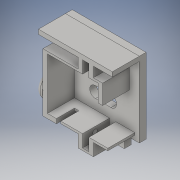
# Autodesk Inventor part: Hip_holder_bare_bone
Saved by Autodesk Inventor 2016 (Build 200138000, 138)
## iProperties
Created: 2018-07-11
Part Number: Hip_holder_bare_bone
Material: Generic
Document SubType Name: Modeling
Designer: Attila
Density: 1 g/cm^3
Appearance: Default
Author: Attila
Autodesk Inventor part; units mm, degrees
sketch "Sketch1" plane through (0, 0, 0) normal (0, 0, 1) x (1, 0, 0)
  line L0 (-20, -25) -> (20, -25)
  line L1 (20, -25) -> (20, 25)
  line L2 (20, 25) -> (-20, 25)
  line L3 (-20, 25) -> (-20, -25)
  line L4 (-20, -25) -> (20, 25) construction
  line L5 (20, -25) -> (-20, 25) construction
  point P0 (0, 0)
  dimension "Szelesseg" = 40
  dimension "Magassag" = 50
  constraints: 12 end point, 2 midpoint, 2 parallel, 1 horizontal, 1 perpendicular
  measures "Szelesseg" distance between parallel lines of L1 L3
  measures "Magassag" distance between parallel lines of L0 L2
extrude "Extrusion1" add sketch "Sketch1" along normal blind 3
sketch "Sketch12" plane through (0, 0, 3) normal (0, 0, 1) x (1, 0, 0)
  line L0 (9.3631, -13.3631) -> (5.2631, -13.3631)
  line L1 (5.2631, -13.3631) -> (5.2631, -18.8631)
  line L2 (2.4631, -17.3356) -> (2.4631, -13.3631)
  line L3 (-13.1369, -13.3631) -> (-13.1369, 9.5369)
  line L4 (-13.1369, 9.5369) -> (2.4631, 9.5369)
  line L5 (2.4631, 9.5369) -> (2.4631, 15.0369)
  line L6 (2.4631, 15.0369) -> (5.2631, 15.0369)
  line L7 (5.2631, 15.0369) -> (5.2631, 9.5369)
  line L8 (5.2631, 9.5369) -> (9.3631, 9.5369)
  line L9 (9.3631, 9.5369) -> (9.3631, 1.9369)
  line L10 (7.2631, -14.3631) -> (7.2631, -19.8631)
  line L11 (7.2631, -19.8631) -> (0.4631, -19.8631)
  line L12 (0.4631, -19.8631) -> (0.4631, -14.3631)
  line L13 (-15.1369, -15.3631) -> (-15.1369, 10.5369)
  line L14 (-15.1369, 10.5369) -> (0.4631, 10.5369)
  line L15 (0.4631, 10.5369) -> (0.4631, 15.0369)
  line L16 (7.2631, 15.0369) -> (7.2631, 10.5369)
  line L17 (7.2631, 10.5369) -> (11.3631, 10.5369)
  line L18 (11.3631, 10.5369) -> (11.3631, 3.6471)
  line L19 (7.2631, -14.3631) -> (13.6631, -14.3631)
  line L20 (13.6631, -14.3631) -> (13.6631, -13.3631)
  line L21 (13.6631, -13.3631) -> (9.3631, -13.3631)
  line L22 (-9.1369, -15.3631) -> (-9.1369, -13.3631)
  line L23 (-7.1369, -14.3631) -> (-7.1369, -13.3631)
  line L24 (0.4631, -14.3631) -> (-7.1369, -14.3631)
  line L25 (-9.1369, -15.3631) -> (-15.1369, -15.3631)
  line L26 (2.4631, -13.3631) -> (-7.1369, -13.3631)
  line L27 (-9.1369, -13.3631) -> (-13.1369, -13.3631)
  line L28 (18.3631, 23.3631) -> (18.3631, -23.3631) projected
  line L29 (18.3631, -23.3631) -> (-18.3631, -23.3631) projected
  line L30 (-18.3631, 23.3631) -> (18.3631, 23.3631) projected
  line L31 (2.4631, -17.3356) -> (2.4631, -18.8631)
  line L32 (-16.127, -21.127) -> (16.127, -21.127) projected
  line L33 (2.4631, -18.8631) -> (5.2631, -18.8631)
  line L34 (11.3631, 3.6471) -> (11.3631, 1.9369)
  line L35 (11.3631, 1.9369) -> (9.3631, 1.9369)
  line L36 (-9.1369, -14.3631) -> (-7.1369, -14.3631)
  line L37 (-9.1369, -13.3631) -> (-7.1369, -13.3631)
  line L38 (7.2631, 15.0369) -> (18.3631, 15.0369)
  line L39 (18.3631, 15.0369) -> (18.3631, 17.0369)
  line L40 (18.3631, 17.0369) -> (-18.3631, 17.0369)
  line L41 (-18.3631, 17.0369) -> (-18.3631, 15.0369)
  line L42 (-18.3631, 15.0369) -> (0.4631, 15.0369)
  line L43 (-18.3631, -23.3631) -> (-18.3631, 15.0369)
  line L44 (-18.3631, 17.0369) -> (-18.3631, 23.3631)
  line L45 (-17.1371, 15.0369) -> (-17.1371, 17.0369)
  line L46 (15.6631, 15.0369) -> (15.6631, 17.0369)
  point P0 (19.6785, 0.2929)
  dimension "d83" = 22.5
  dimension "d85" = 2.8
  dimension "d86" = 2.8
  dimension "d87" = 15.6
  dimension "d88" = 15.6
  dimension "d89" = 4.1
  dimension "d90" = 4.1
  dimension "d91" = 7.6
  dimension "d92" = 5.5
  dimension "d95" = 22.9
  dimension "d97" = 2
  dimension "d98" = 2
  dimension "d100" = 2
  dimension "d101" = 2
  dimension "d102" = 2
  dimension "d103" = 4.3
  dimension "d105" = 2
  dimension "d106" = 1
  dimension "d107" = 1
  dimension "d109" = 1
  dimension "d110" = 4
  dimension "d111" = 2
  dimension "d112" = 2
  dimension "d113" = 1
  dimension "d114" = 22.9
  dimension "d125" = 3.5
  dimension "d130" = 4.7
  dimension "d132" = 9
  dimension "d133" = 5.5
  dimension "d139" = 1
  dimension "d181" = 2
  dimension "d182" = 2
  dimension "d185" = 4.5
  dimension "d186" = 1.226
  dimension "d187" = 2.7
  constraints: 86 end point, 26 perpendicular, 12 point on line, 3 horizontal, 1 midpoint, 1 vertical
  measures "d83" distance between parallel lines of L9 L3
  measures "d85" distance between parallel lines of L5 L7
  measures "d86" distance between parallel lines of L2 L1
  measures "d87" distance of L3.end L4.end
  measures "d88" distance of L2.end L3.start
  measures "d89" distance of L8.end L7.end
  measures "d90" distance of L0.start L0.end
  measures "d91" distance of L8.end L9.end
  measures "d92" distance between parallel lines of L6 L8
  measures "d95" distance between parallel lines of L8 L0
  measures "d97" distance between parallel lines of L9 L18
  measures "d98" distance between parallel lines of L7 L16
  measures "d100" distance between parallel lines of L15 L5
  measures "d101" distance between parallel lines of L13 L3
  measures "d102" distance between parallel lines of L10 L1
  measures "d103" distance of L0.start L20.end
  measures "d105" distance between parallel lines of L12 L2
  measures "d106" distance between parallel lines of L17 L8
  measures "d107" distance between parallel lines of L14 L4
  measures "d109" distance between parallel lines of L0 L19
  measures "d110" distance between parallel lines of L3 L22
  measures "d111" distance between parallel lines of L22 L23
  measures "d112" distance between parallel lines of L27 L25
  measures "d113" distance between parallel lines of L26 L24
  measures "d114" distance between parallel lines of L4 L27
  measures "d125" distance between parallel lines of L29 L11
  measures "d130" distance from line of L20.end L28
  measures "d132" distance between parallel lines of L29 L19
  measures "d133" distance between parallel lines of L26 L33
  measures "d139" distance between parallel lines of L33 L11
  measures "d181" distance of L38.end L39.end
  measures "d182" distance of L40.end L41.end
  measures "d185" distance between parallel lines of L17 L38
  measures "d186" distance between parallel lines of L45 L41
  measures "d187" distance between parallel lines of L28 L46
ref_plane "Work Plane6" through (0, 0, 15) normal (0, 0, 1) x (1, 0, 0)
sketch "Sketch14" plane through (0, 0, 15) normal (0, 0, 1) x (1, 0, 0)
  line L0 (-9.1369, -14.3631) -> (0.4631, -14.3631) projected
  line L1 (-9.1369, -14.3631) -> (-9.1369, -13.3631)
  line L2 (-13.1369, -13.3631) -> (2.4631, -13.3631) projected
  line L3 (-7.1369, -13.3631) -> (-7.1369, -14.3631)
  point P0 (0, 0)
  dimension "d136" = 2
  constraints: 4 end point, 3 point on line, 1 parallel, 1 vertical
  measures "d136" distance between parallel lines of L3 L1
extrude "Extrusion5" cut sketch "Sketch14" against normal blind 8
ref_plane "Work Plane5" through (7.0131, -20.8631, 3) normal (1, 0, 0) x (0, 0, -1)
sketch "Sketch17" plane through (7.0131, -20.8631, 3) normal (1, 0, 0) x (0, 0, -1)
  line L0 (0, 0) -> (-12, 0) projected
  line L1 (0, 7.5) -> (-12, 7.5) projected
  line L2 (0, 6.5) -> (-12, 6.5) projected
  line L3 (-12, 7.5) -> (-12, 30.4) construction
  line L4 (-12, 18.95) -> (0, 18.95) construction
  line L5 (0, 37.9) -> (-12, 37.9) construction
  line L6 (0, 31.4) -> (-12, 31.4) construction
  point P0 (3, 20.8631)
  point P1 (-6.5, 5.5)
  point P2 (-6.5, 32.4)
  dimension "d144" = 1
  dimension "d145" = 18.95
  dimension "d146" = 1
  constraints: 2 end point, 1 midpoint, 1 perpendicular, 1 symmetric about line
  measures "d144" distance from line of point (-6.5, 5.5) L2
  measures "d145" distance between parallel lines of L5 L4
  measures "d146" distance from line of L6 point (-6.5, 32.4)
hole "Hole3" at (7.0131, -15.3631, 9.5) at (7.0131, 11.5369, 9.5) direction (-1, 0, 0) diameter 1.778 depth 8 tip angle 118
ref_plane "Work Plane1" through (-15.1369, -14.3631, 5) normal (-1, 0, 0) x (0, 0, 1)
sketch "Sketch18" plane through (-15.1369, -14.3631, 5) normal (-1, 0, 0) x (0, 0, 1)
  line L0 (9, 0) -> (0, 0) projected
  line L1 (-2, -9) -> (-2, 37.7262) projected
  circle A0 centre (3.9, 6.9) radius 3.6
  circle A1 centre (3.9, 6.9) radius 5.1
  point P0 (-5, 14.3631)
  dimension "d156" = 6.9
  dimension "d157" = 5.9
  dimension "d158" = 7.2
  dimension "d159" = 10.2
  constraints: 2 centre point, 2 coincident
  measures "d156" distance from line of L0 point (3.9, 6.9)
  measures "d157" distance from line of L1 point (3.9, 6.9)
  measures "d158" diameter of A0
  measures "d159" diameter of A1
extrude "Extrusion6" add sketch "Sketch18" along normal blind 4
sketch "Sketch22" plane through (0, 0, 3) normal (0, 0, 1) x (1, 0, 0)
  line L0 (9.0131, -16.3631) -> (15.6631, -16.3631) projected
  line L1 (15.6631, -16.3631) -> (15.6631, 25)
  line L2 (20, 25) -> (-20, 25) projected
  line L3 (9.0131, -22.8631) -> (9.0131, -16.3631) projected
  line L4 (9.0131, -16.3631) -> (9.0131, -22.8631)
  line L5 (-1.5369, -16.3631) -> (-1.5369, -22.8631) projected
  line L6 (9.0131, -22.8631) -> (-1.5369, -22.8631)
  line L7 (-1.5369, -22.8631) -> (-1.5369, -16.3631)
  line L8 (-7.1369, -16.3631) -> (-1.5369, -16.3631) projected
  line L9 (-1.5369, -16.3631) -> (-7.1369, -16.3631)
  line L10 (-17.1369, -17.3631) -> (-7.1369, -17.3631) projected
  line L11 (-7.1369, -17.3631) -> (-7.1369, -16.3631)
  line L12 (-17.1369, -17.3631) -> (-17.1369, 25)
  line L13 (-20, 25) -> (-20, -25)
  line L14 (-20, -25) -> (20, -25)
  line L15 (20, -25) -> (20, 25) projected
  line L16 (20, -25) -> (20, 25)
  line L17 (20, 25) -> (15.6631, 25)
  point P0 (0, 0)
  constraints: 22 end point, 5 collinear, 4 perpendicular, 2 point on line, 2 vertical
extrude "Extrusion7" cut sketch "Sketch22" against normal blind 10 contours L0 L1 L2 L15 L14 L13 L12 L10 L11 L8 L5 L6 L3
ref_plane "Work Plane4" through (-15.1369, -14.3631, 3) normal (-1, 0, 0) x (0, 0, 1)
sketch "Sketch24" plane through (-15.1369, -14.3631, 3) normal (-1, 0, 0) x (0, 0, 1)
  circle A0 centre (5.9, 6.9) radius 5 projected
  line L0 (5.9, 11.9) -> (0, 11.9)
  line L1 (0, -1) -> (0, 24.9) projected
  line L2 (5.9, 1.9) -> (0, 1.9)
  point P0 (-3, 14.3631)
  point P1 (0, 0)
  point P2 (0, 23.9)
  constraints: 4 end point, 2 point on circle, 2 point on line, 2 tangent, 1 horizontal, 1 parallel
extrude "Extrusion8" add sketch "Sketch24" along normal blind 2 contours A0 L2 L1 L0
fillet "Fillet15" radius 1.7 1 edges at (-19.1369, -7.4631, 3.8)
ref_plane "Work Plane3" through (13.6631, -14.3631, 3) normal (1, 0, 0) x (0, 0, -1)
sketch "Sketch30" plane through (13.6631, -14.3631, 3) normal (1, 0, 0) x (0, 0, -1)
  arc A0 (-12, 1) -> (-11, 0) centre (-11, 1) ccw projected
  line L0 (0, 13.7) -> (0, 0.1) projected
  line L1 (-12, 1) -> (0, 1)
  line L2 (0, 1) -> (0, 0)
  line L3 (0, 0) -> (-12, 0)
  line L4 (-12, 0) -> (-12, 1)
  point P0 (3, 14.3631)
  constraints: 8 end point, 2 parallel, 1 horizontal, 1 perpendicular
extrude "Extrusion10" cut sketch "Sketch30" against normal blind 2.3
extrude "Extrusion12" add sketch "Sketch12" along normal blind 12 contours L21 L20 L19 L10 L11 L12 L24 L23 L26 L2 L31 L33 L1 L0 | L22 L25 L13 L14 L15 L42 L45 L40 L46 L38 L16 L17 L18 L34 L35 L9 L8 L7 L6 L5 L4 L3 L27
sketch "Sketch32" plane through (0, 0, 3) normal (0, 0, 1) x (1, 0, 0)
  line L0 (-17.1369, 25) -> (-17.1369, 17.0369) projected
  line L1 (15.6631, 25) -> (-17.1369, 25)
  line L2 (-17.1369, 25) -> (-17.1369, 17.037)
  line L3 (-17.1369, 17.037) -> (15.6631, 17.037)
  line L4 (15.6631, 17.037) -> (15.6631, 25)
  point P0 (0, 0)
  dimension "d190" = 7.963
  constraints: 8 end point, 2 parallel, 1 horizontal, 1 perpendicular, 1 point on line
  measures "d190" distance of L2.end L1.end
extrude "Extrusion13" cut sketch "Sketch32" against normal blind 12
sketch "Sketch33" plane through (7.2631, -19.8631, 3) normal (1, 0, 0) x (0, 0, -1)
  line L0 (0, -3) -> (0, 3.5) projected
  line L1 (0, 5.5) -> (-12, 5.5) projected
  line L2 (0, 3.5) -> (0, 34.9) projected
  line L3 (0, 30.4) -> (-12, 30.4) projected
  point P0 (3, 19.8631)
  point P1 (-6.5, 4.5)
  point P2 (-6.5, 31.4)
  dimension "d194" = 6.5
  dimension "d195" = 1
  dimension "d196" = 6.5
  dimension "d197" = 1
  measures "d194" distance from line of L0 point (-6.5, 4.5)
  measures "d195" distance from line of L1 point (-6.5, 4.5)
  measures "d196" distance from line of L2 point (-6.5, 31.4)
  measures "d197" distance from line of L3 point (-6.5, 31.4)
hole "Hole4" at (7.2631, -15.3631, 9.5) at (7.2631, 11.5369, 9.5) direction (-1, 0, 0) diameter 2 depth 8 tip angle 118
sketch "Sketch35" plane through (0, 0, 3) normal (0, 0, 1) x (1, 0, 0)
  line L0 (-9.1369, -15.3631) -> (-9.1369, -13.3631) projected
  line L1 (0.4631, -14.3631) -> (-7.1369, -14.3631) projected
  line L2 (-9.1369, -13.3631) -> (-7.1369, -13.3631)
  line L3 (-7.1369, -13.3631) -> (-7.1369, -14.3631)
  line L4 (-7.1369, -14.3631) -> (-9.1369, -14.3631)
  line L5 (-9.1369, -14.3631) -> (-9.1369, -13.3631)
  point P0 (0, 0)
  constraints: 8 end point, 2 parallel, 1 horizontal, 1 perpendicular
extrude "Extrusion14" add sketch "Sketch35" along normal blind 4
sketch "Sketch36" plane through (0, 0, 3) normal (0, 0, 1) x (1, 0, 0)
  line L0 (-1.5369, -22.8631) -> (-1.5369, -16.3631) projected
  line L1 (9.0131, -16.3631) -> (9.0131, -22.8631) projected
  line L2 (-1.5369, -22.8631) -> (9.0131, -22.8631)
  line L3 (9.0131, -22.8631) -> (9.0131, -21.8631)
  line L4 (9.0131, -21.8631) -> (-1.5369, -21.8631)
  line L5 (-1.5369, -21.8631) -> (-1.5369, -22.8631)
  point P0 (0, 0)
  dimension "d207" = 1
  constraints: 8 end point, 2 parallel, 1 horizontal, 1 perpendicular, 1 point on line
  measures "d207" distance of L3.end L2.end
extrude "Extrusion15" cut sketch "Sketch36" against normal blind 10
sketch "Sketch41" plane through (0, 0, 0) normal (0, 0, -1) x (-1, 0, 0)
  line L0 (-13.4433, -1.75) -> (-13.4433, 1.75)
  line L1 (-13.4433, 1.75) -> (-12.2074, 1.75)
  line L2 (-12.2074, 1.75) -> (-12.2074, 0.4426)
  line L3 (-12.2074, 0.4426) -> (-8.9151, 0.4426)
  line L4 (-8.9151, 0.4426) -> (-8.9151, 1.75)
  line L5 (-8.9151, 1.75) -> (-7.6724, 1.75)
  line L6 (-7.6724, 1.75) -> (-7.6724, -1.75)
  line L7 (-7.6724, -1.75) -> (-8.9151, -1.75)
  line L8 (-8.9151, -1.75) -> (-8.9151, -0.303)
  line L9 (-8.9151, -0.303) -> (-12.2074, -0.303)
  line L10 (-12.2074, -0.303) -> (-12.2074, -1.75)
  line L11 (-12.2074, -1.75) -> (-13.4433, -1.75)
  line L12 (-4.5027, 1.144) -> (-4.5027, -1.0997)
  line L13 (-4.5027, -1.0997) -> (-1.9424, -1.0997)
  line L14 (-1.9424, -1.0997) -> (-1.9424, 1.144)
  line L15 (-1.9424, 1.144) -> (-0.8563, 1.144)
  line L16 (-0.8563, 1.144) -> (-0.8563, -1.0282)
  spline S0 degree 2 poles (-0.8563, -1.0282) (-0.8563, -1.4402) (-1.3261, -1.75) (-1.9424, -1.75) knots 0 0 0 1 2 2 2
  line L17 (-1.9424, -1.75) -> (-4.5027, -1.75)
  spline S1 degree 2 poles (-4.5027, -1.75) (-5.1155, -1.75) (-5.5751, -1.4436) (-5.5751, -1.0282) knots 0 0 0 1 2 2 2
  line L18 (-5.5751, -1.0282) -> (-5.5751, 1.144)
  line L19 (-5.5751, 1.144) -> (-4.5027, 1.144)
  line L20 (5.6296, 1.0146) -> (2.3373, 1.0146)
  line L21 (2.3373, 1.0146) -> (2.3373, -0.9839)
  line L22 (2.3373, -0.9839) -> (5.6296, -0.9839)
  line L23 (5.6296, -0.9839) -> (5.6296, -0.3643)
  line L24 (5.6296, -0.3643) -> (3.8354, -0.3643)
  line L25 (3.8354, -0.3643) -> (3.8354, 0.3405)
  line L26 (3.8354, 0.3405) -> (6.8349, 0.3405)
  line L27 (6.8349, 0.3405) -> (6.8349, -0.8852)
  spline S2 degree 2 poles (6.8349, -0.8852) (6.8349, -1.3823) (6.3037, -1.75) (5.5956, -1.75) knots 0 0 0 1 2 2 2
  line L28 (5.5956, -1.75) -> (2.3407, -1.75)
  spline S3 degree 2 poles (2.3407, -1.75) (1.6291, -1.75) (1.1014, -1.3823) (1.1014, -0.8852) knots 0 0 0 1 2 2 2
  line L29 (1.1014, -0.8852) -> (1.1014, 0.8886)
  spline S4 degree 2 poles (1.1014, 0.8886) (1.1014, 1.3789) (1.6291, 1.75) (2.3407, 1.75) knots 0 0 0 1 2 2 2
  line L30 (2.3407, 1.75) -> (5.5956, 1.75)
  spline S5 degree 2 poles (5.5956, 1.75) (6.2969, 1.75) (6.8349, 1.3857) (6.8349, 0.9193) knots 0 0 0 1 2 2 2
  line L31 (6.8349, 0.9193) -> (6.8349, 0.7831)
  line L32 (6.8349, 0.7831) -> (5.6296, 0.6401)
  line L33 (5.6296, 0.6401) -> (5.6296, 1.0146)
  spline S6 degree 2 poles (8.7449, 0.429) (8.7449, 0.8375) (9.2011, 1.144) (9.8174, 1.144) knots 0 0 0 1 2 2 2
  line L34 (9.8174, 1.144) -> (12.8101, 1.144)
  spline S7 degree 2 poles (12.8101, 1.144) (13.4297, 1.144) (13.8825, 0.8375) (13.8825, 0.429) knots 0 0 0 1 2 2 2
  line L35 (13.8825, 0.429) -> (13.8825, -1.0282)
  spline S8 degree 2 poles (13.8825, -1.0282) (13.8825, -1.447) (13.4195, -1.75) (12.8101, -1.75) knots 0 0 0 1 2 2 2
  line L36 (12.8101, -1.75) -> (9.8174, -1.75)
  spline S9 degree 2 poles (9.8174, -1.75) (9.2011, -1.75) (8.7449, -1.447) (8.7449, -1.0282) knots 0 0 0 1 2 2 2
  line L37 (8.7449, -1.0282) -> (8.7449, 0.429)
  line L38 (9.8242, -1.0895) -> (12.8033, -1.0895)
  line L39 (12.8033, -1.0895) -> (12.8033, 0.5039)
  line L40 (12.8033, 0.5039) -> (9.8242, 0.5039)
  line L41 (9.8242, 0.5039) -> (9.8242, -1.0895)
  point P0 (0, 0)
  point P1 (0, 0)
  constraints: 1 coincident, 1 other
extrude "Extrusion18" cut sketch "Sketch41" against normal blind 0.5
fillet "Fillet38" radius 1.3 2 edges at (-15.1369, -3.5175, 12.1315) (-15.1369, -11.4087, 12.1315)
fillet "Fillet39" radius 1.3 2 edges at (-17.1369, -2.4631, 5.4475) (-17.1369, -12.4631, 5.4475)
fillet "Fillet40" [suppressed]
sketch "Sketch43" plane through (0, 0, 0) normal (0, 0, -1) x (-1, 0, 0)
  line L0 (-5.5688, 6.5) -> (6.3624, 6.5) construction
  line L1 (-3.0688, 4) -> (3.8624, 4)
  line L2 (3.8624, 9) -> (-3.0688, 9)
  arc A0 (-3.0688, 9) -> (-3.0688, 4) centre (-3.0688, 6.5) ccw
  arc A1 (3.8624, 4) -> (3.8624, 9) centre (3.8624, 6.5) ccw
  line L3 (-5.5688, -6.5) -> (6.3624, -6.5) construction
  line L4 (8.7449, -1.0282) -> (8.7449, 0.429) projected
  line L5 (-3.0688, -9) -> (3.8624, -9)
  line L6 (3.8624, -4) -> (-3.0688, -4)
  arc A2 (-3.0688, -4) -> (-3.0688, -9) centre (-3.0688, -6.5) ccw
  arc A3 (3.8624, -9) -> (3.8624, -4) centre (3.8624, -6.5) ccw
  point P0 (0, 0)
  point P1 (0.3968, 6.5)
  point P2 (0.3968, -6.5)
  dimension "d267" = 5
  dimension "d268" = 5
  dimension "d269" = 4
  dimension "d270" = 4
  constraints: 16 end point, 12 point on circle, 8 tangent, 4 centre point, 4 point on line, 2 midpoint, 2 parallel, 1 horizontal, 1 perpendicular
  measures "d267" diameter of A1
  measures "d268" diameter of A3
  measures "d269" distance from line of L1 point (0, 0)
  measures "d270" distance from line of L6 point (0, 0)
extrude "Extrusion20" cut sketch "Sketch43" against normal blind 10
equation "\"d86\" = d85"
equation "\"d90\" = d89"
equation "\"d95\" = d82"
equation "\"d9\" = 0.5 * d10"
equation "\"d12\" = d11"
equation "\"d13\" = d11"
equation "\"d14\" = d11"
equation "\"d93\" = d92"
equation "\"d82\" = 22.9"
equation "\"d10\" = 18.133333"
equation "\"d11\" = 2"
body "Solid1"
